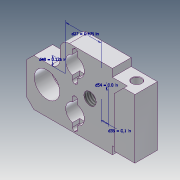
# Autodesk Inventor part: J005822
Saved by Autodesk Inventor 2015 SP1 (Build 190203100, 203)
## iProperties
Created: 2016-08-29
Material: ALUMINUM, 6061-T651
Vendor: HHMI: JRC - ID&F
Document SubType Name: Modeling
Designer: ARNOLDJ
Density: 2.7 g/cm^3
Appearance: Metal-AL-6061 (Machined)
Part Number: J005822
Description: ANGLE ADJ UPPER
Project: P-260102
RuleStatus: InUse
AfterDocSave0: file://Part Number Cleaner
LAB/DEPT: HANTMAN (LAB)
REQUESTING SCIENTIST: HANTMAN, ADAM
SURFACE ROUGHNESS: 63 Ra
DESIGN DEPARTMENT: HHMI: JRC - ID&F
SPECIAL FINISH: NONE
ALTERED ITEM PART NUMBER: N/A
ALTERED ITEM VENDOR: N/A
ALTERED ITEM DESCRIPTION: N/A
Author: ARNOLDJ
Revision Number: -
Autodesk Inventor part; units mm, degrees
ref_plane "YZ Plane" through (0, 0, 0) normal (1, 0, 0) x (0, 1, 0)
ref_plane "XZ Plane" through (0, 0, 0) normal (0, 1, 0) x (-1, 0, 0)
ref_plane "XY Plane" through (0, 0, 0) normal (0, 0, 1) x (1, 0, 0)
sketch "Sketch1" plane through (0, 0, 0) normal (0, 0, 1) x (1, 0, 0)
  line L0 (0, 17.78) -> (0, -17.78) projected
  line L1 (-26.67, 0) -> (26.67, 0) projected
  line L2 (19.05, -12.7) -> (-19.05, -12.7)
  line L3 (-19.05, -12.7) -> (-19.05, 12.7)
  line L4 (-19.05, 12.7) -> (19.05, 12.7)
  line L5 (19.05, 12.7) -> (19.05, -12.7)
  line L6 (19.05, -12.7) -> (-19.05, 12.7) construction
  line L7 (-19.05, -12.7) -> (19.05, 12.7) construction
  point P0 (0, 0)
  dimension "d0" = 25.4
  dimension "d1" = 38.1
  constraints: 12 end point, 2 midpoint, 2 parallel, 1 horizontal, 1 perpendicular
  measures "d0" distance of L2.end L3.end
  measures "d1" distance of L3.end L4.end
extrude "Extrusion1" add sketch "Sketch1" along normal blind 6.35
sketch "Sketch2" plane through (0, 0, 0) normal (0, 0, 1) x (1, 0, 0)
  line L0 (0, 4.445) -> (0, -4.445) projected
  line L1 (-14.986, 0) -> (5.461, 0) projected
  point P0 (0, 0)
  point P1 (2.54, 0)
  point P2 (-12.065, -3.175)
  dimension "d27" = 12.065
  dimension "d35" = 2.54
  dimension "d48" = 3.175
  dimension "d54" = 0
  measures "d27" distance from line of L0 point (-12.065, -3.175)
  measures "d35" distance from line of L0 point (2.54, 0)
  measures "d48" distance from line of point (-12.065, -3.175) L1
  measures "d54" distance from line of L1 point (2.54, 0)
hole "Hole1" at (2.54, 0, 0) direction (0, 0, 1) diameter 4.1402 end through all
sketch "Sketch4" plane through (-19.05, 12.7, 6.35) normal (0, 1, 0) x (1, 0, 0)
  line L0 (19.05, 15.24) -> (19.05, -2.54) projected
  line L1 (45.72, 6.35) -> (-7.62, 6.35) projected
  line L2 (38.1, 6.35) -> (38.1, 0) projected
  line L3 (38.1, 0) -> (0, 0) projected
  point P0 (19.05, 6.35)
  point P1 (34.29, 3.175)
  point P2 (38.1, 12.7)
  dimension "d36" = 3.81
  dimension "d37" = 3.175
  measures "d36" distance from line of point (34.29, 3.175) L2
  measures "d37" distance from line of point (34.29, 3.175) L3
hole "Hole2" at (15.24, 12.7, 3.175) direction (0, -1, 0) diameter 3.175 end through all
hole "Hole3" at (-12.065, -3.175, 0) direction (0, 0, 1) diameter 8.636 end through all counterbore diameter 9.525 counterbore depth 0.635
sketch "Sketch5" plane through (0, 0, 6.35) normal (0, 0, 1) x (1, 0, 0)
  line L0 (19.05, -12.7) -> (19.05, 12.7) projected
  line L1 (19.05, 12.7) -> (-19.05, 12.7) projected
  line L2 (-19.05, -12.7) -> (19.05, -12.7) projected
  line L3 (19.05, 12.7) -> (12.065, 12.7)
  line L4 (12.065, 12.7) -> (12.065, -12.7)
  line L5 (12.065, -12.7) -> (19.05, -12.7)
  line L6 (19.05, -12.7) -> (19.05, 12.7)
  circle A0 centre (2.54, 0) radius 2.0701 projected
  point P0 (0, 0)
  dimension "d39" = 6.985
  dimension "d40" = 9.525
  constraints: 8 end point, 2 parallel, 1 horizontal, 1 perpendicular, 1 point on line
  measures "d39" distance between parallel lines of L0 L4
  measures "d40" distance from line of L4 A0.centre
extrude "Extrusion3" add sketch "Sketch5" along normal blind 1.27 contours L2 L4 L1 L0
sketch "Sketch6" plane through (0, 0, 0) normal (0, 0, 1) x (1, 0, 0)
  line L0 (0, 13.335) -> (0, -13.335) projected
  line L1 (-26.67, 0) -> (26.67, 0) projected
  line L2 (12.065, 12.7) -> (-19.05, 12.7) projected
  line L3 (-19.05, -12.7) -> (12.065, -12.7) projected
  line L4 (19.05, -12.7) -> (19.05, 12.7) projected
  line L5 (19.05, 12.7) -> (10.16, 12.7)
  line L6 (10.16, 12.7) -> (10.16, 10.0838)
  line L7 (10.16, 10.0838) -> (19.05, 10.0838)
  line L8 (19.05, 10.0838) -> (19.05, 12.7)
  line L9 (19.05, -12.7) -> (10.16, -12.7)
  line L10 (10.16, -12.7) -> (10.16, -10.0838)
  line L11 (10.16, -10.0838) -> (19.05, -10.0838)
  line L12 (19.05, -10.0838) -> (19.05, -12.7)
  point P0 (0, 0)
  dimension "d43" = 2.6162
  dimension "d44" = 2.6162
  dimension "d45" = 8.89
  constraints: 16 end point, 4 parallel, 2 horizontal, 2 perpendicular, 1 point on line
  measures "d43" distance of L5.end L6.end
  measures "d44" distance of L9.end L10.end
  measures "d45" distance of L6.end L7.end
extrude "Extrusion4" cut sketch "Sketch6" along normal up to next contours L2 L5 L4 L7 L6 | L10 L11 L4 L9 L3
sketch "Sketch7" plane through (0, 0, 6.35) normal (0, 0, 1) x (1, 0, 0)
  line L0 (-19.05, 12.7) -> (-19.05, -12.7) projected
  line L1 (10.16, 12.7) -> (-19.05, 12.7) projected
  line L2 (-19.05, 12.7) -> (-7.62, 12.7)
  line L3 (-7.62, 12.7) -> (-7.62, 3.175)
  line L4 (-7.62, 3.175) -> (-19.05, 3.175)
  line L5 (-19.05, 3.175) -> (-19.05, 12.7)
  point P0 (0, 0)
  dimension "d49" = 9.525
  dimension "d50" = 11.43
  constraints: 8 end point, 2 parallel, 1 horizontal, 1 perpendicular
  measures "d49" distance between parallel lines of L1 L4
  measures "d50" distance of L3.end L4.end
extrude "Extrusion5" cut sketch "Sketch7" against normal up to next
fillet "Fillet2" radius 3.175 1 edges at (-7.62, 3.175, 3.175)
chamfer "Chamfer1" distance 2.54 angle 45 1 edges at (-19.05, 3.175, 3.175)
chamfer "Chamfer2" distance 2.54 angle 45 1 edges at (-19.05, -12.7, 3.175)
chamfer "Chamfer3" distance 3.175 angle 45 1 edges at (12.065, 10.0838, 6.985)
fillet "Fillet3" radius 3.175 1 edges at (-7.62, 12.7, 3.175)
sketch "Sketch8" plane through (0, 0, 6.35) normal (0, 0, 1) x (1, 0, 0)
  line L0 (0, 17.78) -> (0, -17.78) projected
  line L1 (-26.67, 0) -> (26.67, 0) projected
  point P0 (0, 0)
  point P1 (-2.54, 6.985)
  point P2 (-2.54, -6.985)
  dimension "d69" = 13.97
  dimension "d70" = 6.985
  dimension "d71" = 2.54
  constraints: 1 vertical alignment
  measures "d69" distance of point (-2.54, -6.985) point (-2.54, 6.985)
  measures "d70" distance from line of point (-2.54, 6.985) L1
  measures "d71" distance from line of point (-2.54, 6.985) L0
hole "Hole4" at (-2.54, -6.985, 6.35) at (-2.54, 6.985, 6.35) direction (0, 0, -1) diameter 6.35 end through all
sketch "Sketch9" plane through (0, 0, 6.35) normal (0, 0, 1) x (1, 0, 0)
  circle A0 centre (-2.54, 6.985) radius 3.175 projected
  circle A1 centre (-2.54, -6.985) radius 3.175 projected
  line L0 (-1.651, 1.778) -> (-3.429, 1.778)
  line L1 (-3.429, 1.778) -> (-3.429, 12.192)
  line L2 (-3.429, 12.192) -> (-1.651, 12.192)
  line L3 (-1.651, 12.192) -> (-1.651, 1.778)
  line L4 (-1.651, 1.778) -> (-3.429, 12.192) construction
  line L5 (-3.429, 1.778) -> (-1.651, 12.192) construction
  line L6 (-1.651, -12.192) -> (-3.429, -12.192)
  line L7 (-3.429, -12.192) -> (-3.429, -1.778)
  line L8 (-3.429, -1.778) -> (-1.651, -1.778)
  line L9 (-1.651, -1.778) -> (-1.651, -12.192)
  line L10 (-1.651, -12.192) -> (-3.429, -1.778) construction
  line L11 (-3.429, -12.192) -> (-1.651, -1.778) construction
  point P0 (0, 0)
  dimension "d79" = 10.414
  dimension "d80" = 1.778
  dimension "d81" = 10.414
  dimension "d82" = 1.778
  constraints: 24 end point, 4 midpoint, 4 parallel, 2 horizontal, 2 perpendicular
  measures "d79" distance of L0.end L1.end
  measures "d80" distance of L1.end L2.end
  measures "d81" distance of L6.end L7.end
  measures "d82" distance of L7.end L8.end
extrude "Extrusion6" cut sketch "Sketch9" against normal blind 2.54 contours L3 A0 L1 | A0 L1 L2 L3 | L3 L0 L1 A0 | L9 A1 L7 | A1 L7 L8 L9 | L9 L6 L7 A1
fillet "Fillet4" radius 0.7937 8 edges at (-1.651, -12.192, 5.08) (-3.429, -12.192, 5.08) (-1.651, -1.778, 5.08) (-3.429, -1.778, 5.08) (-1.651, 1.778, 5.08) (-3.429, 1.778, 5.08) (-1.651, 12.192, 5.08) (-3.429, 12.192, 5.08)
chamfer "Chamfer4" distance 1.27 angle 45 1 edges at (-19.05, -4.7625, 0)
chamfer "Chamfer5" distance 0.889 angle 45 2 edges at (-2.54, -3.81, 0) (-2.54, 10.16, 0)
chamfer "Chamfer6" distance 0.127 angle 45 2 edges at (15.24, -10.0838, 1.5875) (15.24, 10.0838, 1.5875)
equation "\"d44\" = d43"
body "Solid1"
